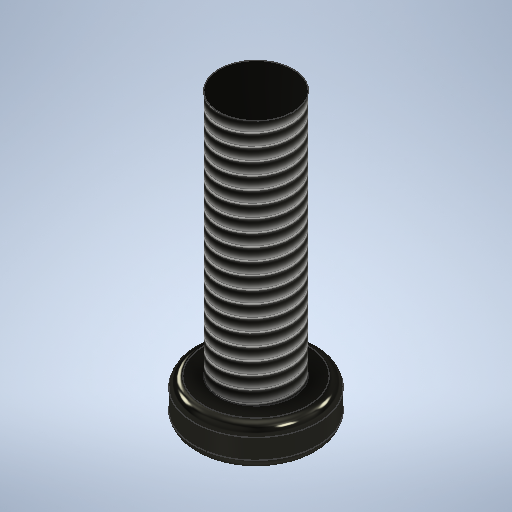
# Autodesk Inventor part: M3 x 10
Saved by Autodesk Inventor 2025.1 (Build 291241000, 241)
## iProperties
Created: 2025-05-06
Part Number: M3 x 10
Material: Generic
Document SubType Name: Modeling
Designer: santiago
Density: 1 g/cm^3
Appearance: Default
Author: santiago
Autodesk Inventor part; units mm, degrees
ref_plane "YZ Plane" through (0, 0, 0) normal (1, 0, 0) x (0, 1, 0)
ref_plane "XZ Plane" through (0, 0, 0) normal (0, 1, 0) x (-1, 0, 0)
ref_plane "XY Plane" through (0, 0, 0) normal (0, 0, 1) x (1, 0, 0)
sketch "Sketch1" plane through (0, 0, 0) normal (0, 1, 0) x (-1, 0, 0)
  circle A0 centre (0, 0) radius 2.5
  dimension "d0" = 5
  constraints: 1 centre point, 1 coincident
  measures "d0" diameter of A0
extrude "Extrusion1" add sketch "Sketch1" along normal blind 1.6
sketch "Sketch2" plane through (0, 1.6, 0) normal (0, 1, 0) x (1, 0, 0)
  circle A0 centre (0, 0) radius 1.5
  dimension "d3" = 3
  constraints: 1 centre point, 1 coincident
  measures "d3" diameter of A0
extrude "Extrusion2" add sketch "Sketch2" along normal blind 10
thread "Thread1" size "M3x0.5" class "6g" standard "ANSI Metric M Profile" full length
fillet "Fillet1" radius 0.4 2 edges at (2.5, 1.6, 0) (2.5, 0, 0)
sketch "Sketch3" plane through (0, 0, 0) normal (0, -1, 0) x (1, 0, 0)
  line L0 (0.0034, 1.75) -> (0.0034, -1.75) construction
  line L1 (-0.5966, 1.15) -> (-0.5966, -1.15)
  line L2 (0.6034, -1.15) -> (0.6034, 1.15)
  arc A0 (0.6034, 1.15) -> (-0.5966, 1.15) centre (0.0034, 1.15) ccw
  arc A1 (-0.5966, -1.15) -> (0.6034, -1.15) centre (0.0034, -1.15) ccw
  line L3 (-1.75, 0.0034) -> (1.75, 0.0034) construction
  line L4 (-1.15, -0.5966) -> (1.15, -0.5966)
  line L5 (1.15, 0.6034) -> (-1.15, 0.6034)
  arc A2 (-1.15, 0.6034) -> (-1.15, -0.5966) centre (-1.15, 0.0034) ccw
  arc A3 (1.15, -0.5966) -> (1.15, 0.6034) centre (1.15, 0.0034) ccw
  point P0 (0, 0)
  point P1 (0.0034, 0)
  point P2 (0.6034, 0)
  point P3 (0, 0.6034)
  point P4 (0, 0.0034)
  point P5 (0.6034, 0.6034)
  point P6 (-0.5966, 0.6034)
  point P7 (-0.5966, -0.5966)
  point P8 (0.6034, -0.5966)
  dimension "d9" = 3.5
  dimension "d10" = 1.2
  dimension "d13" = 90
  constraints: 16 end point, 12 point on circle, 4 centre point, 4 point on line, 4 tangent, 2 midpoint, 1 horizontal alignment, 1 parallel, 1 vertical, 16 other
  measures "d9" distance of L0.start L0.end
  measures "d10" diameter of A1
extrude "Extrusion3" cut sketch "Sketch3" against normal blind 0.8
fillet "Fillet2" radius 0.2 28 edges at (0.6034, 0.4, 0.6034) (0.6034, 0.4, -0.5966) (-0.5966, 0.4, 0.6034) (-0.5966, 0.4, -0.5966) (0.0034, 0, -1.75) (0.6034, 0, -0.8733) (-0.5966, 0, -0.8733) (1.75, 0, 0.0034) (0.8767, 0, 0.6034) (0.8767, 0, -0.5966) (0.0034, 0, 1.75) (-0.5966, 0, 0.8767) (0.6034, 0, 0.8767) (-1.75, 0, 0.0034) (-0.8733, 0, -0.5966) (-0.8733, 0, 0.6034) (0.0034, 0.8, 1.75) (0.6034, 0.8, 0.8767) (-0.5966, 0.8, 0.8767) (1.75, 0.8, 0.0034) (0.8767, 0.8, -0.5966) (0.8767, 0.8, 0.6034) (0.0034, 0.8, -1.75) (0.6034, 0.8, -0.8733) (-0.5966, 0.8, -0.8733) (-1.75, 0.8, 0.0034) (-0.8733, 0.8, -0.5966) (-0.8733, 0.8, 0.6034)
body "Solid1"
